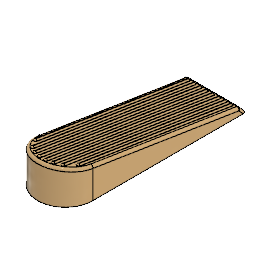
Door Stop (Autodesk Fusion 360 design; units mm, degrees)
Autodesk Fusion 360 part; units mm, degrees
box "BoxPrimitive1" add length 127 width 45.72 height 5.08 placed x (0, 1, 0) y (-1, 0, 0) z (0, 0, 1) at (0, 0, 0)
cylinder "CylinderPrimitive1" add diameter 45.72 height -5.08 placed x (1, 0, 0) y (0, 1, 0) z (0, 0, 1) at (-22.86, 0, 5.08)
draft "Draft1" angle 9 neutral plane through (0, 127, 0) pull (0, 1, 0) 1 faces at (-15.24, 42.3333, 5.08)
chamfer "Chamfer1" distance 5.08 angle 45 1 edges at (-22.86, 127, 5.08)
shell "Shell1" thickness 2.54 removed faces 2 at (-15.24, 127, 0.0003) at (-30.48, 42.3333, 0)
fillet "Fillet1" radius 2.032 6 edges at (-45.72, 60.9913, 15.5348) (-22.86, -22.86, 28.8155) (0, 60.9913, 15.5348) (-22.86, 121.9825, 5.8747) (-45.72, 124.4913, 2.9373) (0, 124.4913, 2.9373)
sketch "Sketch5" plane through (0, 3.8928, 24.5783) normal (0, 0.156434, 0.987688) x (-1, 0, 0)
  line L0 (43.688, -118.8121) -> (43.688, 3.6195)
  ellipse E0 centre (22.86, 3.6195) end of major axis (22.86, 24.7071) minor radius 20.828 (43.688, 3.6195) -> (2.032, 3.6195) ccw
  line L1 (2.032, 3.6195) -> (2.032, -118.8121)
  line L2 (2.032, -118.8121) -> (43.688, -118.8121)
  line L3 (6.35, -116.84) -> (6.35, 31.3132)
  line L4 (6.35, 31.3132) -> (3.81, 31.3132)
  line L5 (3.81, 31.3132) -> (3.81, -116.84)
  arc A0 (3.81, -116.84) -> (6.35, -116.84) centre (5.08, -116.84) ccw
  line L6 (11.43, 31.3132) -> (8.89, 31.3132)
  line L7 (11.43, -116.84) -> (11.43, 31.3132)
  line L8 (8.89, 31.3132) -> (8.89, -116.84)
  arc A1 (8.89, -116.84) -> (11.43, -116.84) centre (10.16, -116.84) ccw
  line L9 (16.51, 31.3132) -> (13.97, 31.3132)
  line L10 (16.51, -116.84) -> (16.51, 31.3132)
  line L11 (13.97, 31.3132) -> (13.97, -116.84)
  arc A2 (13.97, -116.84) -> (16.51, -116.84) centre (15.24, -116.84) ccw
  line L12 (21.59, 31.3132) -> (19.05, 31.3132)
  line L13 (21.59, -116.84) -> (21.59, 31.3132)
  line L14 (19.05, 31.3132) -> (19.05, -116.84)
  arc A3 (19.05, -116.84) -> (21.59, -116.84) centre (20.32, -116.84) ccw
  circle A4 centre (5.08, 10.9427) radius 1.27
  circle A5 centre (10.16, 18.5756) radius 1.27
  circle A6 centre (15.24, 21.59) radius 1.27
  circle A7 centre (20.32, 22.86) radius 1.27
  line L15 (22.86, -118.8121) -> (22.86, -52.353) construction
  line L16 (24.13, -116.84) -> (24.13, 31.3132)
  line L17 (36.83, 31.3132) -> (36.83, -116.84)
  arc A8 (39.37, -116.84) -> (41.91, -116.84) centre (40.64, -116.84) ccw
  arc A9 (24.13, -116.84) -> (26.67, -116.84) centre (25.4, -116.84) ccw
  arc A10 (34.29, -116.84) -> (36.83, -116.84) centre (35.56, -116.84) ccw
  arc A11 (29.21, -116.84) -> (31.75, -116.84) centre (30.48, -116.84) ccw
  line L18 (43.688, 3.6195) -> (43.688, -118.8121)
  line L19 (34.29, -116.84) -> (34.29, 31.3132)
  circle A12 centre (25.4, 22.86) radius 1.27
  line L20 (34.29, 31.3132) -> (36.83, 31.3132)
  line L21 (41.91, 31.3132) -> (41.91, -116.84)
  line L22 (24.13, 31.3132) -> (26.67, 31.3132)
  circle A13 centre (30.48, 21.59) radius 1.27
  circle A14 centre (35.56, 18.5756) radius 1.27
  line L23 (29.21, 31.3132) -> (31.75, 31.3132)
  line L24 (39.37, -116.84) -> (39.37, 31.3132)
  line L25 (31.75, 31.3132) -> (31.75, -116.84)
  line L26 (29.21, -116.84) -> (29.21, 31.3132)
  line L27 (39.37, 31.3132) -> (41.91, 31.3132)
  circle A15 centre (40.64, 10.9427) radius 1.27
  line L28 (26.67, 31.3132) -> (26.67, -116.84)
  point P0 (45.72, 0)
  dimension "d25" = 2.54
  constraint vertical L3
  constraint horizontal L4
  constraint vertical L5
  constraint tangent L5 A4
  constraint tangent L3 A4
  constraint tangent L8 A5
  constraint tangent L7 A5
  constraint tangent L11 A6
  constraint tangent L10 A6
  constraint tangent L14 A7
  constraint tangent L13 A7
  constraint vertical L15
  constraint midpoint L2 L15.start
  constraint symmetric origin L15 P0
  constraint symmetric L1.start L15 L0.end
  constraint symmetric L1.end L15 L0.start
  constraint symmetric L5.end L15 A8.end
  constraint symmetric L3.start L15 A8.start
  constraint symmetric L3.end L15 L24.end
  constraint symmetric L4.end L15 L21.start
  constraint symmetric A0 L15 A8
  constraint symmetric L6.start L15 L19.end
  constraint symmetric L6.end L15 L17.start
  constraint symmetric L7.start L15 A10.start
  constraint symmetric L8.end L15 L17.end
  constraint symmetric A1 L15 A10
  constraint symmetric L9.start L15 L23.start
  constraint symmetric L9.end L15 L23.end
  constraint symmetric L10.start L15 A11.start
  constraint symmetric L11.end L15 A11.end
  constraint symmetric A2 L15 A11
  constraint symmetric L12.start L15 L16.end
  constraint symmetric L12.end L15 L22.end
  constraint symmetric L13.start L15 L16.start
  constraint symmetric L14.end L15 A9.end
  constraint symmetric A3 L15 A9
  constraint symmetric A4 L15 A15
  constraint symmetric A5 L15 A14
  constraint symmetric A6 L15 A13
  constraint symmetric A7 L15 A12
  measures "d25" distance of L5.end L3.start
extrude "Extrude1" add sketch "Sketch5" along normal blind 1.27 contours A15 | A8 L21 L24 A15 | L3 L5 A0 A4 | A4 | A14 | L17 A10 L19 A14 | L7 L8 A1 A5 | A5 | A13 | A11 A13 L25 L26 | L10 L11 A2 A6 | A6 | A12 | L16 A9 A12 L28 | L13 L14 A3 A7 | A7
fillet "Fillet2" radius 1.016 32 edges at (-6.35, 56.3882, 17.5496) (-5.08, -7.9709, 27.7431) (-3.81, 56.3882, 17.5496) (-5.08, 120.7474, 7.3562) (-8.89, 52.6188, 18.1467) (-10.16, 120.7474, 7.3562) (-11.43, 52.6188, 18.1467) (-10.16, -15.5097, 28.9372) (-16.51, 51.1298, 18.3825) (-15.2396, -18.4871, 29.4087) (-13.97, 51.1301, 18.3824) (-15.24, 120.7474, 7.3562) (-21.59, 50.5033, 18.4817) (-20.3203, -19.7414, 29.6074) (-19.05, 50.503, 18.4818) (-20.32, 120.7474, 7.3562) (-26.67, 50.503, 18.4818) (-25.4003, -19.7414, 29.6074) (-24.13, 50.5026, 18.4818) (-25.4, 120.7474, 7.3562) (-31.75, 51.1301, 18.3824) (-30.4804, -18.4871, 29.4087) (-29.21, 51.1298, 18.3825) (-30.48, 120.7474, 7.3562) (-36.83, 52.6188, 18.1467) (-35.56, -15.5097, 28.9372) (-34.29, 52.6188, 18.1467) (-35.56, 120.7474, 7.3562) (-41.91, 56.3882, 17.5496) (-40.64, -7.9709, 27.7431) (-39.37, 56.3882, 17.5496) (-40.64, 120.7474, 7.3562)
